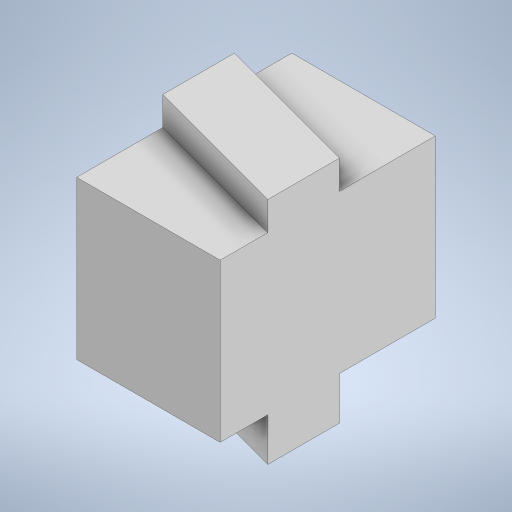
# Autodesk Inventor part: elevator
Saved by Autodesk Inventor 2024 (Build 280153000, 153)
## iProperties
Created: 2025-01-19
Part Number: elevator
Material: Generic
Document SubType Name: Modeling
Designer: domko
Density: 1 g/cm^3
Appearance: Default
Author: domko
Autodesk Inventor part; units mm, degrees
ref_plane "YZ Plane" through (0, 0, 0) normal (1, 0, 0) x (0, 1, 0)
ref_plane "XZ Plane" through (0, 0, 0) normal (0, 1, 0) x (-1, 0, 0)
ref_plane "XY Plane" through (0, 0, 0) normal (0, 0, 1) x (1, 0, 0)
sketch "Sketch1" plane through (0, 0, 0) normal (1, 0, 0) x (0, 1, 0)
  line L0 (6, 13.5008) -> (-5, 13.5008)
  line L1 (-5, 13.5008) -> (-5, -1.4992)
  line L2 (-5, -1.4992) -> (6, -1.4992)
  line L3 (6, -1.4992) -> (6, 13.5008)
  point P0 (0, 0)
  dimension "d0" = 5
  dimension "d1" = 11
  dimension "d2" = 15
  constraints: 8 end point, 2 parallel, 1 horizontal, 1 perpendicular
  measures "d0" distance from line of point (0, 0) L1
  measures "d1" distance of L1.end L2.end
  measures "d2" distance of L0.end L1.end
extrude "Extrusion1" add sketch "Sketch1" along normal blind 10
sketch "Sketch2" plane through (0, -5, -1.4992) normal (0, -1, 0) x (1, 0, 0)
  line L0 (10, 15) -> (10, 0) projected
  line L1 (10, 11.6795) -> (0, 9)
  line L2 (0, 9) -> (0, 4)
  line L3 (0, 15) -> (0, 0) projected
  line L4 (0, 4) -> (10, 6.6795)
  line L5 (10, 6.6795) -> (10, 11.6795)
  line L6 (10, 11.6795) -> (10, 6.6795)
  point P0 (0, 1.4992)
  dimension "d5" = 5
  dimension "d6" = 6
  dimension "d7" = 105
  dimension "d8" = 105
  constraints: 10 end point, 3 point on line, 2 collinear
  measures "d5" distance of L1.end L2.end
  measures "d6" distance of L3.start L1.end
  measures "d7" angle of L1 L2
  measures "d8" angle of L3 L4
extrude "Extrusion2" add sketch "Sketch2" along normal blind 3 and the other way blind 13
body "Solid1"
